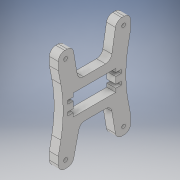
# Autodesk Inventor part: GimbalServoBracket
Saved by Autodesk Inventor 2018 (Build 220112000, 112)
## iProperties
Created: 2019-02-06
Part Number: GimbalServoBracket
Material: Generic
Document SubType Name: Modeling
Designer: anirudh
Density: 1 g/cm^3
Appearance: Default
Author: anirudh
Autodesk Inventor part; units mm, degrees
ref_plane "YZ Plane" through (0, 0, 0) normal (1, 0, 0) x (0, 1, 0)
ref_plane "XZ Plane" through (0, 0, 0) normal (0, 1, 0) x (-1, 0, 0)
ref_plane "XY Plane" through (0, 0, 0) normal (0, 0, 1) x (1, 0, 0)
sketch "Sketch1" plane through (0, 0, 0) normal (1, 0, 0) x (0, 1, 0)
  line L0 (40.477, -40.1066) -> (44.033, -40.1066)
  line L1 (61.051, -82.1182) -> (57.495, -82.1182)
  line L2 (61.051, -40.1066) -> (61.051, -82.1182)
  line L3 (40.477, -82.1182) -> (40.477, -40.1066)
  line L4 (57.495, -86.7114) -> (57.495, -87.503)
  line L5 (54.066, -82.1182) -> (47.462, -82.1182)
  line L6 (57.495, -87.503) -> (54.066, -87.503)
  line L7 (54.066, -87.503) -> (54.066, -82.1182)
  line L8 (54.066, -82.1182) -> (54.138, -82.1182)
  line L9 (57.495, -82.1182) -> (57.495, -87.503)
  line L10 (44.033, -82.1182) -> (40.477, -82.1182)
  line L11 (47.462, -82.1182) -> (47.462, -87.503)
  line L12 (47.462, -82.1182) -> (47.462, -87.503)
  line L13 (47.462, -87.503) -> (44.033, -87.503)
  line L14 (44.033, -87.503) -> (44.033, -82.1182)
  line L15 (44.033, -34.7218) -> (47.462, -34.7218)
  line L16 (47.462, -34.7218) -> (47.462, -40.1066)
  line L17 (44.033, -40.1066) -> (44.033, -34.7218)
  line L18 (47.462, -40.1066) -> (54.138, -40.1066)
  line L19 (57.567, -34.7218) -> (57.567, -40.1066)
  line L20 (57.495, -40.1066) -> (57.567, -40.1066)
  line L21 (57.567, -40.1066) -> (57.567, -34.7218)
  line L22 (57.567, -34.7218) -> (54.138, -34.7218)
  line L23 (54.138, -34.7218) -> (54.138, -40.1066)
  line L24 (40.477, -40.1066) -> (44.033, -40.1066)
  line L25 (47.462, -40.1066) -> (54.138, -40.1066)
  line L26 (57.567, -40.1066) -> (61.051, -40.1066)
  line L27 (44.033, -82.1182) -> (40.477, -82.1182)
  line L28 (61.051, -82.1182) -> (57.495, -82.1182)
  line L29 (54.066, -82.1182) -> (47.462, -82.1182)
  line L30 (101.598, -25.3627) -> (101.598, -34.7099)
  line L31 (101.598, -96.8383) -> (101.598, -87.4911)
  line L32 (101.598, -34.7099) -> (157.1948, -34.7099) construction
  line L33 (69.941, -44.8564) -> (69.941, -77.3684)
  line L34 (31.587, -77.3565) -> (31.587, -46.6047)
  line L35 (0, -25.3627) -> (0, -34.7218)
  line L36 (0, -96.8383) -> (0, -87.503)
  line L37 (101.598, -25.3627) -> (101.598, -34.7099)
  line L38 (101.598, -87.4911) -> (101.598, -96.8383)
  line L39 (0, -96.8383) -> (0, -87.503)
  line L40 (0, -34.7218) -> (0, -25.3627)
  circle A0 centre (7.5, -89.8017) radius 1.85
  circle A1 centre (94.1, -89.8017) radius 1.85
  line L41 (101.598, -87.4911) -> (101.598, -82.7413)
  line L42 (101.598, -82.7413) -> (69.941, -77.3684)
  line L43 (0, -87.503) -> (0, -82.7413)
  line L44 (0, -82.7413) -> (31.587, -77.3565)
  line L45 (0, -96.8383) -> (14.097, -96.8383)
  line L46 (14.097, -96.8383) -> (50.7059, -89.8017)
  line L47 (50.7059, -89.8017) -> (87.3148, -96.8383)
  line L48 (87.3148, -96.8383) -> (101.598, -96.8383)
  line L49 (101.598, -34.7099) -> (101.598, -39.4597)
  line L50 (101.598, -39.4597) -> (69.941, -44.8564)
  line L51 (0, -39.4716) -> (31.587, -46.6047)
  line L52 (0, -34.7218) -> (0, -39.4716)
  circle A2 centre (94.1, -32.4231) radius 1.85
  circle A3 centre (7.5, -32.4231) radius 1.85
  line L53 (101.598, -25.3627) -> (87.3148, -25.3627)
  line L54 (87.3148, -25.3627) -> (50.7059, -32.3992)
  line L55 (50.7059, -32.3992) -> (14.097, -25.3627)
  line L56 (14.097, -25.3627) -> (0, -25.3627)
  point P0 (0, 0)
  constraints: 114 end point, 20 parallel, 10 point on line, 7 horizontal, 7 perpendicular, 4 centre point, 3 vertical
extrude "Extrusion2" add sketch "Sketch1" along normal blind 8.89
fillet "Fillet2" radius 127 2 edges at (4.445, 50.7059, -32.3992) (4.445, 50.7059, -89.8017)
fillet "Fillet3" radius 6.35 12 edges at (4.445, 69.941, -77.3684) (4.445, 69.941, -44.8564) (4.445, 31.587, -46.6047) (4.445, 31.587, -77.3565) (4.445, 101.598, -25.3627) (4.445, 101.598, -39.4597) (4.445, 101.598, -82.7413) (4.445, 101.598, -96.8383) (4.445, 0, -82.7413) (4.445, 0, -96.8383) (4.445, 0, -39.4716) (4.445, 0, -25.3627)
body "Solid2"
